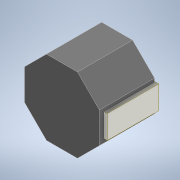
# Autodesk Inventor part: CDRH8D58LD
Saved by Autodesk Inventor 2022 (Build 260153070, 153G)
## iProperties
Created: 2021-11-12
Part Number: CDRH8D58LD
Material: Generic
Document SubType Name: Modeling
Designer: elmar
Density: 1 g/cm^3
Appearance: Default
Author: elmar
Autodesk Inventor part; units mm, degrees
ref_plane "YZ Plane" through (0, 0, 0) normal (1, 0, 0) x (0, 1, 0)
ref_plane "XZ Plane" through (0, 0, 0) normal (0, 1, 0) x (-1, 0, 0)
ref_plane "XY Plane" through (0, 0, 0) normal (0, 0, 1) x (1, 0, 0)
sketch "Sketch1" plane through (0, 0, 0) normal (0, 0, 1) x (1, 0, 0)
  line L0 (-1.6569, 4) -> (1.6569, 4)
  line L1 (1.6569, 4) -> (4, 1.6569)
  line L2 (4, 1.6569) -> (4, -1.6569)
  line L3 (4, -1.6569) -> (1.6569, -4)
  line L4 (1.6569, -4) -> (-1.6569, -4)
  line L5 (-1.6569, -4) -> (-4, -1.6569)
  line L6 (-4, -1.6569) -> (-4, 1.6569)
  line L7 (-4, 1.6569) -> (-1.6569, 4)
  point P0 (0, 0)
  point P1 (0, 0)
  dimension "d0" = 8
  constraints: 16 end point, 1 coincident, 1 horizontal, 17 other
  measures "d0" distance between parallel lines of L0 L4
extrude "Extrusion1" add sketch "Sketch1" along normal blind 6
sketch "Sketch2" plane through (0, 0, 0) normal (0, 0, -1) x (-1, 0, 0)
  line L0 (-3.15, -1.25) -> (-4.35, -1.25)
  line L1 (-4.35, -1.25) -> (-4.35, 1.25)
  line L2 (-4.35, 1.25) -> (-3.15, 1.25)
  line L3 (-3.15, 1.25) -> (-3.15, -1.25)
  line L4 (-3.15, -1.25) -> (-4.35, 1.25) construction
  line L5 (-4.35, -1.25) -> (-3.15, 1.25) construction
  line L6 (3.15, -1.25) -> (4.35, -1.25)
  line L7 (4.35, -1.25) -> (4.35, 1.25)
  line L8 (4.35, 1.25) -> (3.15, 1.25)
  line L9 (3.15, 1.25) -> (3.15, -1.25)
  line L10 (3.15, -1.25) -> (4.35, 1.25) construction
  line L11 (4.35, -1.25) -> (3.15, 1.25) construction
  line L12 (0, -5.6) -> (0, 5.6) projected
  line L13 (6.09, 0) -> (-6.09, 0) projected
  point P0 (0, 0)
  point P1 (-3.75, 0)
  point P2 (3.75, 0)
  point P3 (-3.75, 0)
  point P4 (3.75, 0)
  dimension "d3" = 6.3
  dimension "d4" = 1.2
  dimension "d5" = 2.5
  constraints: 24 end point, 6 midpoint, 4 parallel, 2 equal length, 2 horizontal, 2 perpendicular, 2 point on line, 1 other
  measures "d3" distance between parallel lines of L9 L3
  measures "d4" distance of L1.end L2.end
  measures "d5" distance of L6.end L7.end
extrude "Extrusion2" add sketch "Sketch2" against normal blind 5.5 separate body
thicken "Thicken1" operation add thickness 0.1 both sides no extend neighbours yes toward (0, 0, 1) bodies 1 faces at (-0.2288, 0.5523, 0)
body "Solid1"
body "Solid2"
